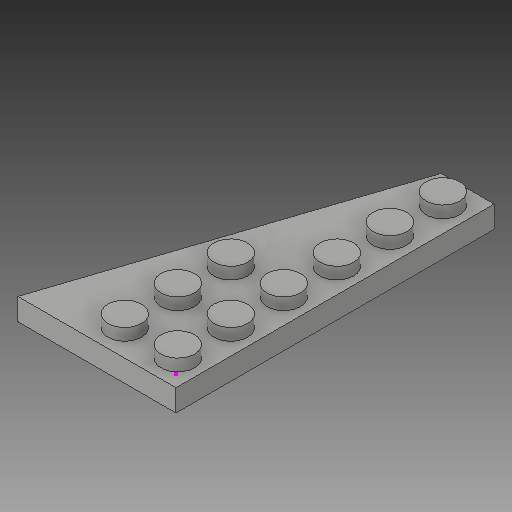
# Autodesk Inventor part: opposite grey peice
Saved by Autodesk Inventor 2017 (Build 210142000, 142)
## iProperties
Created: 2018-05-14
Part Number: opposite grey peice
Material: Generic
Document SubType Name: Modeling
Designer: 19000369
Density: 1 g/cm^3
Appearance: Light Gray
Mass: 1.74968 g
Surface Area: 27.8727 cm^2
Volume: 1.74968 cm^3
Author: 19000369
Autodesk Inventor part; units mm, degrees
ref_plane "YZ Plane" through (0, 0, 0) normal (1, 0, 0) x (0, 1, 0)
ref_plane "XZ Plane" through (0, 0, 0) normal (0, 1, 0) x (-1, 0, 0)
sketch "Sketch1" plane through (0, 0, 0) normal (0, 1, 0) x (-1, 0, 0)
  line L0 (0, 0) -> (0, -47.0662)
  line L1 (0, -47.0662) -> (7.8486, -47.0662)
  line L2 (0, 0) -> (23.3934, 0)
  line L3 (23.3934, 0) -> (7.8486, -47.0662)
  dimension "d0" = 47.0662
  dimension "d1" = 7.8486
  dimension "d2" = 23.3934
  constraints: 8 end point, 2 horizontal, 1 vertical
  measures "d0" distance of L0.start L0.end
  measures "d1" distance of L0.end L1.end
  measures "d2" distance of L0.start L2.end
extrude "Extrusion1" add sketch "Sketch1" along normal blind 3.236
sketch "Sketch2" plane through (0, 3.236, 0) normal (0, 1, 0) x (1, 0, 0)
  circle A0 centre (-3.6594, 3.9218) radius 2.4879
  line L0 (-23.3934, 0) -> (0, 0) projected
  dimension "d5" = 4.9759
  dimension "d6" = 3.9218
  constraints: 1 centre point
  measures "d5" diameter of A0
  measures "d6" distance from line of L0 A0.centre
extrude "Extrusion2" add sketch "Sketch2" along normal blind 1.7577
ref_plane "Work Plane1" through (-11.503, 4.9936, -43.1394) normal (0, 1, 0) x (1, 0, 0)
sketch "Sketch3" plane through (-11.503, 4.9936, -43.1394) normal (0, 1, 0) x (1, 0, 0)
  point P0 (11.503, -43.1394)
pattern_linear "Rectangular Pattern2" count 6 spacing 7.8435 along (0, 0, -1) of "Extrusion2"
pattern_linear "Rectangular Pattern3" count 2 spacing 7.8435 along (-1, 0, 0) of "Extrusion2"
pattern_linear "Rectangular Pattern4" count 3 spacing 7.8435 along (0, 0, -1) of "Extrusion2", "Rectangular Pattern3"
shell "Shell1" thickness 1.4732 removed faces 1 at (-10.414, 0, -15.6887)
sketch "Sketch5" plane through (-21.3554, 1.7628, -1.4732) normal (0, -1, 0) x (1, 0, 0)
  circle A0 centre (14.3004, -14.2138) radius 2.4879
  circle A1 centre (14.3004, -22.0574) radius 2.4879
  circle A2 centre (14.3004, -29.9009) radius 2.4879
  circle A3 centre (14.3004, -14.2138) radius 3.2245
  circle A4 centre (14.3004, -22.0574) radius 3.2245
  circle A5 centre (14.3004, -29.9009) radius 3.2245
  circle A6 centre (6.4569, -6.3703) radius 2.4879
  circle A7 centre (6.4569, -6.3703) radius 3.2245
  circle A8 centre (14.3004, -6.3703) radius 2.4879
  circle A9 centre (14.3004, -6.3703) radius 3.2245
  line L0 (-2.038, 1.4732) -> (21.3554, 1.4732) projected
  line L1 (14.5717, -44.1198) -> (0, 0) projected
  line L2 (5.7322, -17.3559) -> (5.4452, -16.4868)
  line L3 (4.2905, -12.9906) -> (4.0034, -12.1215)
  arc A10 (5.7322, -17.3559) -> (4.0034, -12.1215) centre (6.4569, -14.2138) ccw
  arc A11 (5.4452, -16.4868) -> (4.2905, -12.9906) centre (6.4569, -14.2138) ccw
  line L4 (13.4975, -40.8674) -> (13.2036, -39.9775)
  line L5 (12.0893, -36.6039) -> (11.7954, -35.714)
  arc A12 (13.4975, -40.8674) -> (11.7954, -35.714) centre (14.3004, -37.7444) ccw
  arc A13 (13.2036, -39.9775) -> (12.0893, -36.6039) centre (14.3004, -37.7444) ccw
  dimension "d38" = 4.9759
  dimension "d39" = 4.9759
  dimension "d40" = 4.9759
  dimension "d42" = 6.4491
  dimension "d43" = 6.4491
  dimension "d45" = 6.4491
  dimension "d46" = 4.9759
  dimension "d47" = 6.4491
  dimension "d49" = 7.8435
  dimension "d50" = 7.8435
  dimension "d55" = 4.9759
  dimension "d56" = 6.4491
  dimension "d57" = 7.8435
  dimension "d58" = 7.8435
  dimension "d59" = 7.8435
  constraints: 14 centre point, 8 end point, 8 point on circle, 8 point on line, 5 coincident, 1 horizontal alignment, 1 vertical alignment
  measures "d38" diameter of A0
  measures "d39" diameter of A1
  measures "d40" diameter of A2
  measures "d42" diameter of A3
  measures "d43" diameter of A4
  measures "d45" diameter of A5
  measures "d46" diameter of A6
  measures "d47" diameter of A7
  measures "d49" distance of A1.centre A0.centre
  measures "d50" distance of A2.centre A1.centre
  measures "d55" diameter of A8
  measures "d56" diameter of A9
  measures "d57" distance from line of L0 A8.centre
  measures "d58" distance of A3.centre A8.centre
  measures "d59" distance of A8.centre A6.centre
extrude "Extrusion5" add sketch "Sketch5" along normal blind 1.7628 contours A3 | A4 | A5 | A7 | A9 | L1 A11 A10 | L1 A13 A12
sketch "Sketch7" plane through (0, 0, 0) normal (0, -1, 0) x (1, 0, 0)
  line L0 (-7.8486, -47.0662) -> (-23.3934, 0) projected
  line L1 (-22.6158, -2.3544) -> (-21.2169, -1.8924)
  line L2 (-17.3519, -13.5947) -> (-21.3554, -1.4732) projected
  line L3 (-21.2169, -1.8924) -> (-19.554, -6.9274)
  line L4 (-19.554, -6.9274) -> (-20.9529, -7.3894)
  line L5 (-22.6158, -2.3544) -> (-20.9529, -7.3894)
  line L6 (-19.9376, -10.4635) -> (-18.5387, -10.0015)
  line L7 (-18.2511, -15.5697) -> (-16.8522, -15.1077)
  line L8 (-16.8522, -15.1077) -> (-18.5387, -10.0015)
  line L9 (-19.9376, -10.4635) -> (-18.2511, -15.5697)
  line L10 (-13.7932, -29.0674) -> (-12.3943, -28.6053)
  line L11 (-12.3943, -28.6053) -> (-10.7022, -33.7286)
  line L12 (-9.5599, -37.1872) -> (-15.6232, -18.8291) projected
  line L13 (-12.1011, -34.1907) -> (-13.7932, -29.0674)
  line L14 (-12.1011, -34.1907) -> (-10.7022, -33.7286)
  line L15 (-11.4016, -36.3084) -> (-10.0028, -35.8464)
  line L16 (-10.0028, -35.8464) -> (-8.3101, -40.9713)
  line L17 (-8.1518, -41.4507) -> (-9.266, -38.0771) projected
  line L18 (-9.709, -41.4333) -> (-8.3101, -40.9713)
  line L19 (-9.709, -41.4333) -> (-11.4016, -36.3084)
  point P0 (0, 0)
  constraints: 32 end point, 6 point on line, 3 perpendicular, 1 collinear, 1 parallel, 17 other
extrude "Extrusion6" cut sketch "Sketch7" against normal blind 1.7577 contours L0 L6 L2 L8 L7 | L0 L15 L12 L16 L18 | L0 L10 L11 L14 | L0 L1 L2 L4
body "Solid1"
